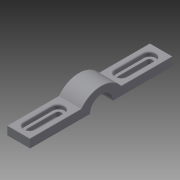
# Autodesk Inventor part: holder
Saved by Autodesk Inventor 2015 (Build 190159000, 159)
## iProperties
Created: 2015-09-29
Part Number: holder
Material: Generic
Document SubType Name: Modeling
Designer: Ross
Density: 1 g/cm^3
Appearance: Default
Author: Ross
Autodesk Inventor part; units mm, degrees
ref_plane "YZ Plane" through (0, 0, 0) normal (1, 0, 0) x (0, 1, 0)
ref_plane "XZ Plane" through (0, 0, 0) normal (0, 1, 0) x (-1, 0, 0)
ref_plane "XY Plane" through (0, 0, 0) normal (0, 0, 1) x (1, 0, 0)
sketch "Sketch1" plane through (0, 0, 0) normal (1, 0, 0) x (0, 1, 0)
  point P0 (0, 0)
sketch "Sketch2" plane through (0, 0, 0) normal (1, 0, 0) x (0, 1, 0)
  line L0 (0, 25) -> (3, 25)
  arc A0 (0, 4) -> (0, 4) centre (0, 0.0048) ccw
  line L1 (3, 25) -> (3, 7)
  line L2 (6.5079, 0) -> (4, 0)
  arc A1 (6.5079, 0) -> (3, 7) centre (-2.2302, 0) ccw
  arc A2 (4, 0) -> (0, 4) centre (0, 0) ccw
  line L3 (0, 4) -> (0, 25)
  point P0 (0, 0)
  dimension "d0" = 25
  dimension "d1" = 3
  dimension "d2" = 4
  dimension "d5" = 18
  dimension "d22" = 4
  constraints: 8 end point, 6 point on circle, 3 centre point, 2 vertical
  measures "d0" distance of point (0, 0) L0.start
  measures "d1" distance of L0.start L0.end
  measures "d2" distance of point (0, 0) A0.end
  measures "d5" distance of L0.end L1.end
  measures "d22" radius of A2
extrude "Extrusion1" add sketch "Sketch2" along normal blind 8 contours L0 L1 A1 L2 A2 L3
sketch "Sketch3" plane through (0, 3, 25) normal (0, 1, 0) x (1, 0, 0)
  line L0 (0, 0) -> (8, 0)
  line L1 (8, 0) -> (4, 0)
  line L2 (4, 0) -> (4, 21)
  line L3 (4, 21) -> (0, 21)
  line L4 (0, 21) -> (4, 21)
  line L5 (8, 21) -> (0, 21) projected
  line L6 (4, 0) -> (4, 2)
  line L7 (4, 2) -> (4, 4)
  circle A0 centre (4, 4) radius 2
  line L8 (0, 18) -> (8, 18) projected
  line L9 (4, 18) -> (4, 14)
  circle A1 centre (4, 14) radius 2
  line L10 (2, 4) -> (2, 14)
  line L11 (6, 4) -> (6, 14)
  point P0 (0, 25)
  dimension "d10" = 2
  dimension "d11" = 2
  dimension "d12" = 4
  dimension "d13" = 4
  constraints: 20 end point, 5 point on circle, 3 point on line, 2 centre point, 2 coincident, 2 midpoint, 2 tangent, 1 collinear, 1 horizontal, 1 perpendicular, 1 vertical
  measures "d10" distance of L1.end L6.end
  measures "d11" distance of L6.end L7.end
  measures "d12" distance of L9.start L9.end
  measures "d13" diameter of A1
extrude "Extrusion2" cut sketch "Sketch3" against normal blind 1.5
sketch "Sketch4" plane through (0, 1.5, 25) normal (0, 1, 0) x (1, 0, 0)
  arc A0 (6, 14) -> (2, 14) centre (4, 14) ccw projected
  line L0 (2, 14) -> (4, 14)
  line L1 (4, 14) -> (6, 14)
  line L2 (6, 14) -> (6, 4)
  arc A1 (2, 4) -> (6, 4) centre (4, 4) ccw projected
  line L3 (6, 4) -> (2, 4)
  line L4 (2, 4) -> (2, 14)
  line L5 (2, 4) -> (2, 14) projected
  circle A2 centre (4, 4) radius 1
  line L6 (4, 4) -> (4, 14)
  line L7 (0, 0) -> (8, 0) projected
  circle A3 centre (4, 14) radius 1
  line L8 (3, 4) -> (3, 14)
  line L9 (5, 4) -> (5, 14)
  point P0 (0, 25)
  dimension "d16" = 2
  dimension "d17" = 2
  constraints: 16 end point, 4 point on circle, 4 tangent, 3 perpendicular, 2 centre point, 2 coincident, 2 collinear, 2 midpoint, 2 point on line, 1 horizontal
  measures "d16" diameter of A2
  measures "d17" diameter of A3
extrude "Extrusion3" cut sketch "Sketch4" against normal blind 1.5 contours A3 L6 L1 | L1 L0 A3 | L9 A2 L6 A3 | L0 L6 A3 | A3 L6 A2 L8 | A2 L3 | L3 L6 A2 | A2 L6 L3
fillet "Fillet1" radius 0.5 4 edges at (6, 3, 16) (4, 3, 23) (2, 3, 16) (4, 3, 9)
fillet "Fillet2" radius 0.2 4 edges at (5, 1.5, 16) (4, 1.5, 22) (3, 1.5, 16) (4, 1.5, 10)
sketch "Sketch5" plane through (0, 0, 0) normal (0, 0, 1) x (1, 0, 0)
  point P0 (0, 0)
mirror "Mirror1" about plane through (0, 0, 0) normal (0, 0, 1)
fillet "Fillet3" radius 0.2 1 edges at (0, 3, -16)
fillet "Fillet4" radius 0.2 2 edges at (4, 3, -25) (0, 1.5, -25)
fillet "Fillet5" radius 0.2 7 edges at (8, 1.5, -25) (8, 3, -16) (8, 5.5819, 3.9149) (0, 5.5819, 3.9149) (8, 3, 16) (4, 3, 25) (0, 3, 16)
body "Solid1"
